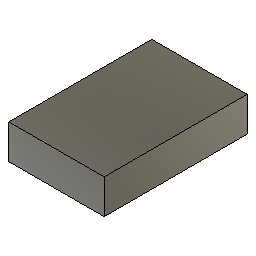
matek h743 v1 (Autodesk Fusion 360 design; units mm, degrees)
Autodesk Fusion 360 part; units mm, degrees
sketch "Sketch1" plane through (0, 0, 0) normal (0, 0, 1) x (1, 0, 0)
  line L0 (18, -27) -> (-18, -27)
  line L1 (-18, -27) -> (-18, 27)
  line L2 (-18, 27) -> (18, 27)
  line L3 (18, 27) -> (18, -27)
  line L4 (18, -27) -> (-18, 27) construction
  line L5 (-18, -27) -> (18, 27) construction
  dimension "d1" = 36
  dimension "d2" = 54
  constraint horizontal L0
  constraint perpendicular L0 L1
  constraint parallel L0 L2
  constraint parallel L1 L3
  constraint coincident L4 origin
  constraint coincident L5 origin
  measures "d1" distance of L1.end L2.end
  measures "d2" distance of L0.end L1.end
extrude "Extrude1" add sketch "Sketch1" along normal blind 13
